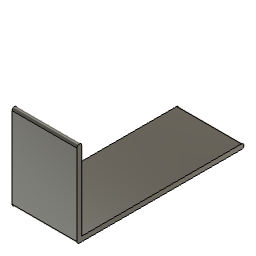
Super Nintendo Bookend (Autodesk Fusion 360 design; units mm, degrees)
Autodesk Fusion 360 part; units mm, degrees
sketch "Sketch1" plane through (0, 0, 0) normal (0, 0, 1) x (1, 0, 0)
  line L0 (0, 0) -> (40, 0)
  line L1 (40, 0) -> (40, 100)
  line L2 (40, 100) -> (0, 100)
  line L3 (0, 100) -> (0, 0)
  line L4 (0, 0) -> (40, 0)
  line L5 (40, 0) -> (40, -3)
  line L6 (40, -3) -> (0, -3)
  line L7 (0, -3) -> (0, 0)
  dimension "d1" = 40
  dimension "d2" = 100
  dimension "d3" = 3
  constraint horizontal L0
  constraint vertical L1
  constraint horizontal L2
  constraint vertical L3
  constraint coincident L0.start L3.end
  constraint horizontal L4
  constraint vertical L5
  constraint horizontal L6
  constraint vertical L7
  measures "d1" distance of L0.start L0.end
  measures "d2" distance of L0.start L2.end
  measures "d3" distance of L0.start L6.end
extrude "Extrude1" add sketch "Sketch1" along normal blind 3 contours L0 L1 L2 L3 L4
extrude "Extrude2" add sketch "Sketch1" along normal blind 53 contours L0 L4 L5 L6 L7
sketch "Sketch2" plane through (0, 0, 0) normal (0, 0, -1) x (1, 0, 0)
  line L0 (0, 3) -> (0, -100)
  line L1 (0, -100) -> (40, -100)
  line L2 (40, -100) -> (40, 3)
  line L3 (40, 3) -> (0, 3)
  line L4 (24.7693, -53.3473) -> (24.431, -53.3473)
  spline S0 degree 3 poles (24.431, -53.3473) (24.2139, -53.3473) (24.1606, -53.2593) (24.1978, -53.0849) knots 0 0 0 0 1 1 1 1
  line L5 (24.1978, -53.0849) -> (24.5069, -51.627)
  spline S1 degree 3 poles (24.5069, -51.627) (24.5472, -51.4375) (24.6658, -51.3707) (24.7869, -51.3707) knots 0 0 0 0 1 1 1 1
  line L6 (24.7869, -51.3707) -> (25.1077, -51.3707)
  spline S2 degree 3 poles (25.1077, -51.3707) (25.2147, -51.3707) (25.2409, -51.4245) (25.2243, -51.5104) knots 0 0 0 0 1 1 1 1
  line L7 (25.2243, -51.5104) -> (24.8804, -53.3006)
  spline S3 degree 3 poles (24.8804, -53.3006) (24.8729, -53.3388) (24.8277, -53.3473) (24.7693, -53.3473) knots 0 0 0 0 1 1 1 1
  line L8 (29.44, -53.3473) -> (29.0786, -53.3473)
  spline S4 degree 3 poles (29.0786, -53.3473) (28.8549, -53.3473) (28.8282, -53.1648) (28.8453, -53.0849) knots 0 0 0 0 1 1 1 1
  line L9 (28.8453, -53.0849) -> (29.1545, -51.621)
  spline S5 degree 3 poles (29.1545, -51.621) (29.1912, -51.4466) (29.2711, -51.3702) (29.347, -51.3702) knots 0 0 0 0 1 1 1 1
  line L10 (29.347, -51.3702) -> (29.7844, -51.3702)
  spline S6 degree 3 poles (29.7844, -51.3702) (29.8879, -51.3702) (29.9186, -51.4199) (29.901, -51.5099) knots 0 0 0 0 1 1 1 1
  line L11 (29.901, -51.5099) -> (29.5511, -53.3001)
  spline S7 degree 3 poles (29.5511, -53.3001) (29.5431, -53.3408) (29.4802, -53.3468) (29.44, -53.3473) knots 0 0 0 0 1 1 1 1
  spline S8 degree 3 poles (3.9225, -53.3709) (3.7023, -53.3709) (3.5566, -53.194) (3.5958, -52.9743) knots 0 0 0 0 1 1 1 1
  line L12 (3.5958, -52.9743) -> (4.2955, -49.0964)
  spline S9 degree 3 poles (4.2955, -49.0964) (4.3353, -48.8772) (4.5363, -48.6942) (4.756, -48.6942) knots 0 0 0 0 1 1 1 1
  spline S10 degree 3 poles (4.756, -48.6942) (4.9762, -48.6942) (5.0692, -48.8767) (5.03, -49.0964) knots 0 0 0 0 1 1 1 1
  line L13 (5.03, -49.0964) -> (4.3363, -52.9743)
  spline S11 degree 3 poles (4.3363, -52.9743) (4.2945, -53.2071) (4.1498, -53.3709) (3.9225, -53.3709) knots 0 0 0 0 1 1 1 1
  line L14 (6.9488, -53.3709) -> (6.605, -53.3709)
  spline S12 degree 3 poles (6.605, -53.3709) (6.3848, -53.3709) (6.231, -53.194) (6.2727, -52.9743) knots 0 0 0 0 1 1 1 1
  line L15 (6.2727, -52.9743) -> (7.0077, -49.0964)
  spline S13 degree 3 poles (7.0077, -49.0964) (7.0494, -48.8767) (7.26, -48.6942) (7.4802, -48.6942) knots 0 0 0 0 1 1 1 1
  line L16 (7.4802, -48.6942) -> (7.8185, -48.6942)
  line L17 (7.8185, -48.6942) -> (6.9498, -53.3709)
  line L18 (6.9498, -53.3709) -> (6.9488, -53.3709)
  spline S14 degree 3 poles (4.383, -54.0531) (4.7027, -54.0531) (5.0084, -53.7902) (5.0652, -53.4639) knots 0 0 0 0 1 1 1 1
  line L19 (5.0652, -53.4639) -> (5.8992, -48.6766)
  spline S15 degree 3 poles (5.8992, -48.6766) (5.9525, -48.371) (5.7509, -48.1287) (5.4442, -48.1287) knots 0 0 0 0 1 1 1 1
  line L20 (5.4442, -48.1287) -> (4.2136, -48.1287)
  spline S16 degree 3 poles (4.2136, -48.1287) (3.9049, -48.1287) (3.6063, -48.3715) (3.549, -48.6766) knots 0 0 0 0 1 1 1 1
  line L21 (3.549, -48.6766) -> (2.6452, -53.4639)
  spline S17 degree 3 poles (2.6452, -53.4639) (2.5838, -53.7902) (2.7924, -54.0531) (3.1122, -54.0531) knots 0 0 0 0 1 1 1 1
  line L22 (3.1122, -54.0531) -> (4.383, -54.0531)
  line L23 (7.5848, -54.0531) -> (8.7103, -48.1287)
  line L24 (8.7103, -48.1287) -> (7.0077, -48.1287)
  spline S18 degree 3 poles (7.0077, -48.1287) (6.6985, -48.1287) (6.4004, -48.3715) (6.3431, -48.6766) knots 0 0 0 0 1 1 1 1
  line L25 (6.3431, -48.6766) -> (5.4392, -53.4639)
  spline S19 degree 3 poles (5.4392, -53.4639) (5.3769, -53.7907) (5.5855, -54.0531) (5.9052, -54.0531) knots 0 0 0 0 1 1 1 1
  line L26 (5.9052, -54.0531) -> (7.5848, -54.0531)
  line L27 (10.5528, -54.0531) -> (11.6783, -48.1287)
  line L28 (11.6783, -48.1287) -> (10.8152, -48.1287)
  line L29 (10.8152, -48.1287) -> (10.1214, -51.5632)
  line L30 (10.1214, -51.5632) -> (9.8475, -48.1287)
  line L31 (9.8475, -48.1287) -> (9.1009, -48.1287)
  line L32 (9.1009, -48.1287) -> (7.9754, -54.0531)
  line L33 (7.9754, -54.0531) -> (8.8385, -54.0531)
  line L34 (8.8385, -54.0531) -> (9.4156, -50.9569)
  line L35 (9.4156, -50.9569) -> (9.8007, -54.0531)
  line L36 (9.8007, -54.0531) -> (10.5528, -54.0531)
  line L37 (12.448, -54.0531) -> (13.6143, -48.1287)
  line L38 (13.6143, -48.1287) -> (11.9754, -48.1287)
  line L39 (11.9754, -48.1287) -> (11.8181, -48.8637)
  line L40 (11.8181, -48.8637) -> (12.6973, -48.8637)
  line L41 (12.6973, -48.8637) -> (12.3022, -50.8639)
  line L42 (12.3022, -50.8639) -> (11.4742, -50.8639)
  line L43 (11.4742, -50.8639) -> (11.3576, -51.4823)
  line L44 (11.3576, -51.4823) -> (12.1856, -51.4823)
  line L45 (12.1856, -51.4823) -> (11.8241, -53.3192)
  line L46 (11.8241, -53.3192) -> (10.9961, -53.3192)
  line L47 (10.9961, -53.3192) -> (10.8649, -54.0531)
  line L48 (10.8649, -54.0531) -> (12.448, -54.0531)
  line L49 (14.5005, -54.0531) -> (14.6403, -53.3182)
  line L50 (14.6403, -53.3182) -> (14.1738, -53.3182)
  line L51 (14.1738, -53.3182) -> (15.0952, -48.1282)
  line L52 (15.0952, -48.1282) -> (14.2436, -48.1282)
  line L53 (14.2436, -48.1282) -> (13.3046, -53.3182)
  line L54 (13.3046, -53.3182) -> (12.8808, -53.3182)
  line L55 (12.8808, -53.3182) -> (12.7395, -54.0531)
  line L56 (12.7395, -54.0531) -> (14.5005, -54.0531)
  line L57 (17.3926, -54.0531) -> (18.5182, -48.1287)
  line L58 (18.5182, -48.1287) -> (17.655, -48.1287)
  line L59 (17.655, -48.1287) -> (16.9613, -51.5632)
  line L60 (16.9613, -51.5632) -> (16.6873, -48.1287)
  line L61 (16.6873, -48.1287) -> (15.9408, -48.1287)
  line L62 (15.9408, -48.1287) -> (14.8152, -54.0531)
  line L63 (14.8152, -54.0531) -> (15.6784, -54.0531)
  line L64 (15.6784, -54.0531) -> (16.2555, -50.9569)
  line L65 (16.2555, -50.9569) -> (16.6406, -54.0531)
  line L66 (16.6406, -54.0531) -> (17.3926, -54.0531)
  line L67 (18.5297, -54.0531) -> (19.6553, -48.1287)
  line L68 (19.6553, -48.1287) -> (18.9088, -48.1287)
  line L69 (18.9088, -48.1287) -> (17.7837, -54.0531)
  line L70 (17.7837, -54.0531) -> (18.5297, -54.0531)
  line L71 (21.4922, -54.0531) -> (22.6178, -48.1287)
  line L72 (22.6178, -48.1287) -> (21.7606, -48.1287)
  line L73 (21.7606, -48.1287) -> (21.0669, -51.5632)
  line L74 (21.0669, -51.5632) -> (20.7929, -48.1287)
  line L75 (20.7929, -48.1287) -> (20.0464, -48.1287)
  line L76 (20.0464, -48.1287) -> (18.9208, -54.0531)
  line L77 (18.9208, -54.0531) -> (19.778, -54.0531)
  line L78 (19.778, -54.0531) -> (20.3611, -50.9569)
  line L79 (20.3611, -50.9569) -> (20.7457, -54.0531)
  line L80 (20.7457, -54.0531) -> (21.4922, -54.0531)
  line L81 (25.4867, -54.0531) -> (26.6062, -48.1287)
  line L82 (26.6062, -48.1287) -> (25.8597, -48.1287)
  line L83 (25.8597, -48.1287) -> (25.3525, -50.8111)
  line L84 (25.3525, -50.8111) -> (24.8216, -50.8111)
  spline S20 degree 3 poles (24.8216, -50.8111) (24.698, -50.8111) (24.6487, -50.6392) (24.7166, -50.2803) knots 0 0 0 0 1 1 1 1
  line L85 (24.7166, -50.2803) -> (25.1248, -48.1287)
  line L86 (25.1248, -48.1287) -> (24.3782, -48.1287)
  line L87 (24.3782, -48.1287) -> (23.9585, -50.4145)
  spline S21 degree 3 poles (23.9585, -50.4145) (23.9032, -50.7141) (24.147, -50.8539) (24.4019, -50.9102) knots 0 0 0 0 1 1 1 1
  spline S22 degree 3 poles (24.4019, -50.9102) (24.1882, -50.9941) (23.7866, -51.1334) (23.7428, -51.3591) knots 0 0 0 0 1 1 1 1
  line L88 (23.7428, -51.3591) -> (23.3346, -53.4639)
  spline S23 degree 3 poles (23.3346, -53.4639) (23.2718, -53.7907) (23.4814, -54.0531) (23.8011, -54.0531) knots 0 0 0 0 1 1 1 1
  line L89 (23.8011, -54.0531) -> (25.4867, -54.0531)
  line L90 (27.4925, -54.0531) -> (28.6588, -48.1287)
  line L91 (28.6588, -48.1287) -> (27.0154, -48.1287)
  line L92 (27.0154, -48.1287) -> (26.8626, -48.8637)
  line L93 (26.8626, -48.8637) -> (27.7409, -48.8637)
  line L94 (27.7409, -48.8637) -> (27.3523, -50.8639)
  line L95 (27.3523, -50.8639) -> (26.5243, -50.8639)
  line L96 (26.5243, -50.8639) -> (26.4077, -51.4823)
  line L97 (26.4077, -51.4823) -> (27.2356, -51.4823)
  line L98 (27.2356, -51.4823) -> (26.8682, -53.3192)
  line L99 (26.8682, -53.3192) -> (26.0402, -53.3192)
  line L100 (26.0402, -53.3192) -> (25.9035, -54.0531)
  line L101 (25.9035, -54.0531) -> (27.4925, -54.0531)
  line L102 (30.1574, -54.0531) -> (31.2829, -48.1287)
  line L103 (31.2829, -48.1287) -> (30.5364, -48.1287)
  line L104 (30.5364, -48.1287) -> (30.0232, -50.8111)
  line L105 (30.0232, -50.8111) -> (29.1183, -50.8111)
  spline S24 degree 3 poles (29.1183, -50.8111) (28.8091, -50.8111) (28.5246, -51.0575) (28.4592, -51.3591) knots 0 0 0 0 1 1 1 1
  line L106 (28.4592, -51.3591) -> (28.0053, -53.4639)
  spline S25 degree 3 poles (28.0053, -53.4639) (27.9359, -53.7892) (28.1521, -54.0531) (28.4723, -54.0531) knots 0 0 0 0 1 1 1 1
  line L107 (28.4723, -54.0531) -> (30.1574, -54.0531)
  line L108 (32.8398, -54.0531) -> (33.8307, -48.6766)
  spline S26 degree 3 poles (33.8307, -48.6766) (33.887, -48.3715) (33.6773, -48.1287) (33.3702, -48.1287) knots 0 0 0 0 1 1 1 1
  line L109 (33.3702, -48.1287) -> (32.2562, -48.1287)
  spline S27 degree 3 poles (32.2562, -48.1287) (31.9475, -48.1287) (31.6514, -48.372) (31.5916, -48.6766) knots 0 0 0 0 1 1 1 1
  line L110 (31.5916, -48.6766) -> (30.5364, -54.0531)
  line L111 (30.5364, -54.0531) -> (31.2362, -54.0531)
  line L112 (31.2362, -54.0531) -> (32.2848, -48.8285)
  spline S28 degree 3 poles (32.2848, -48.8285) (32.2999, -48.7531) (32.3723, -48.6887) (32.4482, -48.6887) knots 0 0 0 0 1 1 1 1
  line L113 (32.4482, -48.6887) -> (33.0022, -48.6887)
  spline S29 degree 3 poles (33.0022, -48.6887) (33.0796, -48.6887) (33.1339, -48.7526) (33.1188, -48.8285) knots 0 0 0 0 1 1 1 1
  line L114 (33.1188, -48.8285) -> (32.0933, -54.0531)
  line L115 (32.0933, -54.0531) -> (32.8398, -54.0531)
  spline S30 degree 3 poles (34.9859, -54.0531) (35.3056, -54.0531) (35.6087, -53.7887) (35.6741, -53.4639) knots 0 0 0 0 1 1 1 1
  line L116 (35.6741, -53.4639) -> (35.9018, -52.3328)
  spline S31 degree 3 poles (35.9018, -52.3328) (35.93, -52.1931) (35.8747, -52.091) (35.8435, -51.9598) knots 0 0 0 0 1 1 1 1
  spline S32 degree 3 poles (35.8435, -51.9598) (35.7696, -51.6497) (34.7325, -50.1913) (34.7707, -49.9711) knots 0 0 0 0 1 1 1 1
  line L117 (34.7707, -49.9711) -> (34.9225, -49.0964)
  spline S33 degree 3 poles (34.9225, -49.0964) (34.9608, -48.8762) (35.1106, -48.6998) (35.3307, -48.6998) knots 0 0 0 0 1 1 1 1
  spline S34 degree 3 poles (35.3307, -48.6998) (35.5509, -48.6998) (35.7033, -48.8762) (35.663, -49.0964) knots 0 0 0 0 1 1 1 1
  line L118 (35.663, -49.0964) -> (35.465, -50.1813)
  line L119 (35.465, -50.1813) -> (36.2457, -50.1813)
  line L120 (36.2457, -50.1813) -> (36.5081, -48.6766)
  spline S35 degree 3 poles (36.5081, -48.6766) (36.5614, -48.371) (36.3548, -48.1287) (36.0476, -48.1287) knots 0 0 0 0 1 1 1 1
  line L121 (36.0476, -48.1287) -> (34.9336, -48.1287)
  spline S36 degree 3 poles (34.9336, -48.1287) (34.6249, -48.1287) (34.3314, -48.3715) (34.2746, -48.6766) knots 0 0 0 0 1 1 1 1
  spline S37 degree 3 poles (34.2746, -48.6766) (34.2228, -48.9577) (33.989, -50.0817) (33.989, -50.1813) knots 0 0 0 0 1 1 1 1
  spline S38 degree 3 poles (33.989, -50.1813) (33.989, -50.2381) (34.0086, -50.2763) (34.0182, -50.2919) knots 0 0 0 0 1 1 1 1
  line L122 (34.0182, -50.2919) -> (35.0447, -52.0006)
  spline S39 degree 3 poles (35.0447, -52.0006) (35.1096, -52.1086) (35.1191, -52.177) (35.1206, -52.269) knots 0 0 0 0 1 1 1 1
  spline S40 degree 3 poles (35.1206, -52.269) (35.1221, -52.3605) (35.0326, -52.7732) (34.998, -52.9748) knots 0 0 0 0 1 1 1 1
  spline S41 degree 3 poles (34.998, -52.9748) (34.9603, -53.195) (34.7516, -53.3714) (34.5314, -53.3714) knots 0 0 0 0 1 1 1 1
  spline S42 degree 3 poles (34.5314, -53.3714) (34.3113, -53.3714) (34.1836, -53.194) (34.2278, -52.9748) knots 0 0 0 0 1 1 1 1
  line L123 (34.2278, -52.9748) -> (34.4264, -52.0011)
  line L124 (34.4264, -52.0011) -> (33.6391, -52.0011)
  line L125 (33.6391, -52.0011) -> (33.3652, -53.4649)
  spline S43 degree 3 poles (33.3652, -53.4649) (33.3038, -53.7902) (33.5114, -54.0531) (33.8312, -54.0531) knots 0 0 0 0 1 1 1 1
  line L126 (33.8312, -54.0531) -> (34.9859, -54.0531)
  line L127 (36.6418, -47.6154) -> (36.6418, -45.6735)
  line L128 (36.6418, -45.6735) -> (3.357, -45.6735)
  line L129 (3.357, -45.6735) -> (3.357, -47.6154)
  line L130 (3.357, -47.6154) -> (36.6418, -47.6154)
  line L131 (35.9189, -47.3646) -> (35.5751, -47.3646)
  line L132 (35.5751, -47.3646) -> (35.5982, -47.2012)
  line L133 (35.5982, -47.2012) -> (35.7847, -47.2012)
  line L134 (35.7847, -47.2012) -> (35.8606, -46.793)
  line L135 (35.8606, -46.793) -> (35.6796, -46.793)
  line L136 (35.6796, -46.793) -> (35.7028, -46.6527)
  line L137 (35.7028, -46.6527) -> (35.8893, -46.6527)
  line L138 (35.8893, -46.6527) -> (35.9591, -46.2099)
  line L139 (35.9591, -46.2099) -> (35.7782, -46.2099)
  line L140 (35.7782, -46.2099) -> (35.8073, -46.0465)
  line L141 (35.8073, -46.0465) -> (36.1803, -46.0465)
  line L142 (36.1803, -46.0465) -> (35.9179, -47.3641)
  line L143 (35.9179, -47.3641) -> (35.9189, -47.3646)
  line L144 (34.3092, -47.3646) -> (34.1459, -47.3646)
  line L145 (34.1459, -47.3646) -> (34.0584, -46.6764)
  line L146 (34.0584, -46.6764) -> (33.9302, -47.3646)
  line L147 (33.9302, -47.3646) -> (33.7377, -47.3646)
  line L148 (33.7377, -47.3646) -> (33.9885, -46.047)
  line L149 (33.9885, -46.047) -> (34.1519, -46.047)
  line L150 (34.1519, -46.047) -> (34.2162, -46.8111)
  line L151 (34.2162, -46.8111) -> (34.3681, -46.047)
  line L152 (34.3681, -46.047) -> (34.5606, -46.047)
  line L153 (34.5606, -46.047) -> (34.3092, -47.3646)
  line L154 (32.5598, -47.3646) -> (32.1747, -47.3646)
  line L155 (32.1747, -47.3646) -> (32.1979, -47.2012)
  line L156 (32.1979, -47.2012) -> (32.2969, -47.2012)
  line L157 (32.2969, -47.2012) -> (32.507, -46.0465)
  line L158 (32.507, -46.0465) -> (32.6935, -46.0465)
  line L159 (32.6935, -46.0465) -> (32.4894, -47.2012)
  line L160 (32.4894, -47.2012) -> (32.5945, -47.2012)
  line L161 (32.5945, -47.2012) -> (32.5598, -47.3646)
  line L162 (30.8632, -47.3646) -> (30.5133, -47.3646)
  line L163 (30.5133, -47.3646) -> (30.5425, -47.2012)
  line L164 (30.5425, -47.2012) -> (30.7234, -47.2012)
  line L165 (30.7234, -47.2012) -> (30.8049, -46.793)
  line L166 (30.8049, -46.793) -> (30.6239, -46.793)
  line L167 (30.6239, -46.793) -> (30.647, -46.6527)
  line L168 (30.647, -46.6527) -> (30.828, -46.6527)
  line L169 (30.828, -46.6527) -> (30.9145, -46.2099)
  line L170 (30.9145, -46.2099) -> (30.7229, -46.2099)
  line L171 (30.7229, -46.2099) -> (30.746, -46.0465)
  line L172 (30.746, -46.0465) -> (31.1191, -46.0465)
  line L173 (31.1191, -46.0465) -> (30.8632, -47.3646)
  line L174 (29.2188, -47.3646) -> (28.8458, -47.3646)
  spline S44 degree 3 poles (28.8458, -47.3646) (28.7764, -47.3646) (28.7332, -47.3032) (28.7468, -47.2304) knots 0 0 0 0 1 1 1 1
  line L175 (28.7468, -47.2304) -> (28.8342, -46.7638)
  spline S45 degree 3 poles (28.8342, -46.7638) (28.8438, -46.7131) (28.9328, -46.6718) (28.98, -46.6527) knots 0 0 0 0 1 1 1 1
  spline S46 degree 3 poles (28.98, -46.6527) (28.9142, -46.6527) (28.8709, -46.6206) (28.881, -46.5653) knots 0 0 0 0 1 1 1 1
  line L176 (28.881, -46.5653) -> (28.9745, -46.0465)
  line L177 (28.9745, -46.0465) -> (29.1439, -46.0465)
  line L178 (29.1439, -46.0465) -> (29.0504, -46.5246)
  spline S47 degree 3 poles (29.0504, -46.5246) (29.0424, -46.5663) (29.0358, -46.6412) (29.0735, -46.6412) knots 0 0 0 0 1 1 1 1
  line L179 (29.0735, -46.6412) -> (29.1902, -46.6412)
  line L180 (29.1902, -46.6412) -> (29.3008, -46.0465)
  line L181 (29.3008, -46.0465) -> (29.4697, -46.0465)
  line L182 (29.4697, -46.0465) -> (29.2188, -47.3646)
  line L183 (27.5508, -47.3646) -> (27.1602, -47.3646)
  line L184 (27.1602, -47.3646) -> (27.1834, -47.2012)
  line L185 (27.1834, -47.2012) -> (27.2824, -47.2012)
  line L186 (27.2824, -47.2012) -> (27.4925, -46.0465)
  line L187 (27.4925, -46.0465) -> (27.679, -46.0465)
  line L188 (27.679, -46.0465) -> (27.4749, -47.2012)
  line L189 (27.4749, -47.2012) -> (27.58, -47.2012)
  line L190 (27.58, -47.2012) -> (27.5508, -47.3646)
  line L191 (25.5948, -47.3646) -> (25.4239, -47.3646)
  line L192 (25.4239, -47.3646) -> (25.4832, -46.047)
  line L193 (25.4832, -46.047) -> (25.6798, -46.047)
  line L194 (25.6798, -46.047) -> (25.6506, -46.3501)
  line L195 (25.6506, -46.3501) -> (25.7848, -46.3501)
  line L196 (25.7848, -46.3501) -> (25.8778, -46.047)
  line L197 (25.8778, -46.047) -> (26.0688, -46.047)
  line L198 (26.0688, -46.047) -> (25.5958, -47.3646)
  line L199 (25.5958, -47.3646) -> (25.5948, -47.3646)
  line L200 (24.058, -47.3646) -> (23.8891, -47.3646)
  line L201 (23.8891, -47.3646) -> (24.14, -46.047)
  line L202 (24.14, -46.047) -> (24.3033, -46.047)
  line L203 (24.3033, -46.047) -> (24.058, -47.3646)
  line L204 (22.5534, -47.3646) -> (22.39, -47.3646)
  line L205 (22.39, -47.3646) -> (22.3026, -46.6764)
  line L206 (22.3026, -46.6764) -> (22.1744, -47.3646)
  line L207 (22.1744, -47.3646) -> (21.9879, -47.3646)
  line L208 (21.9879, -47.3646) -> (22.2327, -46.047)
  line L209 (22.2327, -46.047) -> (22.4016, -46.047)
  line L210 (22.4016, -46.047) -> (22.4745, -46.8111)
  line L211 (22.4745, -46.8111) -> (22.6117, -46.047)
  line L212 (22.6117, -46.047) -> (22.8043, -46.047)
  line L213 (22.8043, -46.047) -> (22.5534, -47.3646)
  line L214 (20.6235, -47.3646) -> (20.4078, -47.3646)
  line L215 (20.4078, -47.3646) -> (20.3727, -46.6005)
  line L216 (20.3727, -46.6005) -> (20.0379, -47.3646)
  line L217 (20.0379, -47.3646) -> (19.8292, -47.3646)
  line L218 (19.8292, -47.3646) -> (20.0519, -46.047)
  line L219 (20.0519, -46.047) -> (20.2153, -46.047)
  line L220 (20.2153, -46.047) -> (20.1102, -46.7407)
  line L221 (20.1102, -46.7407) -> (20.4018, -46.047)
  line L222 (20.4018, -46.047) -> (20.5184, -46.047)
  line L223 (20.5184, -46.047) -> (20.5536, -46.7583)
  line L224 (20.5536, -46.7583) -> (20.6818, -46.047)
  line L225 (20.6818, -46.047) -> (20.8683, -46.047)
  line L226 (20.8683, -46.047) -> (20.6235, -47.3646)
  line L227 (18.5066, -47.3646) -> (18.1572, -47.3646)
  line L228 (18.1572, -47.3646) -> (18.1859, -47.2012)
  line L229 (18.1859, -47.2012) -> (18.3724, -47.2012)
  line L230 (18.3724, -47.2012) -> (18.4483, -46.793)
  line L231 (18.4483, -46.793) -> (18.2673, -46.793)
  line L232 (18.2673, -46.793) -> (18.2904, -46.6527)
  line L233 (18.2904, -46.6527) -> (18.4769, -46.6527)
  line L234 (18.4769, -46.6527) -> (18.5679, -46.2099)
  line L235 (18.5679, -46.2099) -> (18.3658, -46.2099)
  line L236 (18.3658, -46.2099) -> (18.395, -46.0465)
  line L237 (18.395, -46.0465) -> (18.7625, -46.0465)
  line L238 (18.7625, -46.0465) -> (18.5066, -47.3646)
  line L239 (16.8155, -47.3646) -> (16.6521, -47.3646)
  line L240 (16.6521, -47.3646) -> (16.5646, -46.6764)
  line L241 (16.5646, -46.6764) -> (16.4365, -47.3646)
  line L242 (16.4365, -47.3646) -> (16.2499, -47.3646)
  line L243 (16.2499, -47.3646) -> (16.4948, -46.047)
  line L244 (16.4948, -46.047) -> (16.6581, -46.047)
  line L245 (16.6581, -46.047) -> (16.7225, -46.8111)
  line L246 (16.7225, -46.8111) -> (16.8743, -46.047)
  line L247 (16.8743, -46.047) -> (17.0668, -46.047)
  line L248 (17.0668, -46.047) -> (16.8155, -47.3646)
  line L249 (15.0837, -47.3646) -> (14.6931, -47.3646)
  line L250 (14.6931, -47.3646) -> (14.7222, -47.2012)
  line L251 (14.7222, -47.2012) -> (14.8213, -47.2012)
  line L252 (14.8213, -47.2012) -> (15.0254, -46.0465)
  line L253 (15.0254, -46.0465) -> (15.2119, -46.0465)
  line L254 (15.2119, -46.0465) -> (15.0078, -47.2012)
  line L255 (15.0078, -47.2012) -> (15.1128, -47.2012)
  line L256 (15.1128, -47.2012) -> (15.0837, -47.3646)
  line L257 (10.8328, -47.3646) -> (10.6458, -47.3646)
  line L258 (10.6458, -47.3646) -> (10.5834, -46.8629)
  line L259 (10.5834, -46.8629) -> (10.3255, -47.3646)
  line L260 (10.3255, -47.3646) -> (10.1154, -47.3646)
  line L261 (10.1154, -47.3646) -> (10.5467, -46.6005)
  line L262 (10.5467, -46.6005) -> (10.6518, -46.0465)
  line L263 (10.6518, -46.0465) -> (10.8383, -46.0465)
  line L264 (10.8383, -46.0465) -> (10.7222, -46.6412)
  line L265 (10.7222, -46.6412) -> (10.8328, -47.3646)
  line L266 (7.5823, -47.3646) -> (7.1751, -47.3646)
  line L267 (7.1751, -47.3646) -> (7.2057, -47.2012)
  line L268 (7.2057, -47.2012) -> (7.3048, -47.2012)
  line L269 (7.3048, -47.2012) -> (7.5089, -46.0465)
  line L270 (7.5089, -46.0465) -> (7.7014, -46.0465)
  line L271 (7.7014, -46.0465) -> (7.4973, -47.2012)
  line L272 (7.4973, -47.2012) -> (7.6124, -47.2012)
  line L273 (7.6124, -47.2012) -> (7.5823, -47.3646)
  line L274 (6.0374, -47.3646) -> (5.6875, -47.3646)
  line L275 (5.6875, -47.3646) -> (5.7187, -47.2012)
  line L276 (5.7187, -47.2012) -> (5.8997, -47.2012)
  line L277 (5.8997, -47.2012) -> (5.9811, -46.787)
  line L278 (5.9811, -46.787) -> (5.7946, -46.787)
  line L279 (5.7946, -46.787) -> (5.8182, -46.6527)
  line L280 (5.8182, -46.6527) -> (6.0042, -46.6527)
  line L281 (6.0042, -46.6527) -> (6.0927, -46.2094)
  line L282 (6.0927, -46.2094) -> (5.8942, -46.2094)
  line L283 (5.8942, -46.2094) -> (5.9223, -46.046)
  line L284 (5.9223, -46.046) -> (6.2953, -46.046)
  line L285 (6.2953, -46.046) -> (6.0369, -47.3636)
  line L286 (6.0369, -47.3636) -> (6.0374, -47.3646)
  line L287 (4.5992, -47.3646) -> (4.3835, -47.3646)
  line L288 (4.3835, -47.3646) -> (4.3483, -46.6005)
  line L289 (4.3483, -46.6005) -> (4.016, -47.3646)
  line L290 (4.016, -47.3646) -> (3.8059, -47.3646)
  line L291 (3.8059, -47.3646) -> (4.0276, -46.047)
  line L292 (4.0276, -46.047) -> (4.191, -46.047)
  line L293 (4.191, -46.047) -> (4.0859, -46.7407)
  line L294 (4.0859, -46.7407) -> (4.3775, -46.047)
  line L295 (4.3775, -46.047) -> (4.4941, -46.047)
  line L296 (4.4941, -46.047) -> (4.5293, -46.7583)
  line L297 (4.5293, -46.7583) -> (4.6575, -46.047)
  line L298 (4.6575, -46.047) -> (4.85, -46.047)
  line L299 (4.85, -46.047) -> (4.5992, -47.3646)
  line L300 (12.1448, -47.3591) -> (11.8885, -47.3591)
  spline S48 degree 3 poles (11.8885, -47.3591) (11.8191, -47.3591) (11.7718, -47.3038) (11.7834, -47.2309) knots 0 0 0 0 1 1 1 1
  line L301 (11.7834, -47.2309) -> (11.8352, -46.9041)
  line L302 (11.8352, -46.9041) -> (12.0096, -46.9041)
  line L303 (12.0096, -46.9041) -> (11.9704, -47.1198)
  spline S49 degree 3 poles (11.9704, -47.1198) (11.9613, -47.1685) (11.991, -47.2072) (12.0403, -47.2072) knots 0 0 0 0 1 1 1 1
  spline S50 degree 3 poles (12.0403, -47.2072) (12.0895, -47.2072) (12.1363, -47.1685) (12.1453, -47.1198) knots 0 0 0 0 1 1 1 1
  line L304 (12.1453, -47.1198) -> (12.1745, -46.9624)
  spline S51 degree 3 poles (12.1745, -46.9624) (12.1765, -46.9519) (12.1619, -46.9116) (12.1569, -46.9041) knots 0 0 0 0 1 1 1 1
  line L305 (12.1569, -46.9041) -> (11.9121, -46.5251)
  spline S52 degree 3 poles (11.9121, -46.5251) (11.9045, -46.5135) (11.9055, -46.5065) (11.906, -46.5019) knots 0 0 0 0 1 1 1 1
  line L306 (11.906, -46.5019) -> (11.9704, -46.1696)
  spline S53 degree 3 poles (11.9704, -46.1696) (11.9835, -46.1033) (12.0478, -46.047) (12.1162, -46.047) knots 0 0 0 0 1 1 1 1
  line L307 (12.1162, -46.047) -> (12.3781, -46.047)
  spline S54 degree 3 poles (12.3781, -46.047) (12.446, -46.047) (12.4892, -46.1028) (12.4771, -46.1696) knots 0 0 0 0 1 1 1 1
  line L308 (12.4771, -46.1696) -> (12.4188, -46.5019)
  line L309 (12.4188, -46.5019) -> (12.2499, -46.5019)
  line L310 (12.2499, -46.5019) -> (12.2906, -46.2626)
  spline S55 degree 3 poles (12.2906, -46.2626) (12.2992, -46.2139) (12.27, -46.1691) (12.2207, -46.1691) knots 0 0 0 0 1 1 1 1
  spline S56 degree 3 poles (12.2207, -46.1691) (12.1715, -46.1691) (12.1247, -46.2134) (12.1157, -46.2626) knots 0 0 0 0 1 1 1 1
  line L311 (12.1157, -46.2626) -> (12.0805, -46.4552)
  line L312 (12.0805, -46.4552) -> (12.3313, -46.8986)
  spline S57 degree 3 poles (12.3313, -46.8986) (12.3374, -46.9091) (12.3489, -46.9488) (12.3429, -46.98) knots 0 0 0 0 1 1 1 1
  line L313 (12.3429, -46.98) -> (12.2961, -47.2309)
  spline S58 degree 3 poles (12.2961, -47.2309) (12.2806, -47.3153) (12.2449, -47.3591) (12.1448, -47.3591) knots 0 0 0 0 1 1 1 1
  line L314 (8.8963, -47.3591) -> (8.64, -47.3591)
  spline S59 degree 3 poles (8.64, -47.3591) (8.5706, -47.3591) (8.5233, -47.3038) (8.5349, -47.2309) knots 0 0 0 0 1 1 1 1
  line L315 (8.5349, -47.2309) -> (8.5867, -46.9041)
  line L316 (8.5867, -46.9041) -> (8.7611, -46.9041)
  line L317 (8.7611, -46.9041) -> (8.7214, -47.1198)
  spline S60 degree 3 poles (8.7214, -47.1198) (8.7123, -47.1685) (8.742, -47.2072) (8.7913, -47.2072) knots 0 0 0 0 1 1 1 1
  spline S61 degree 3 poles (8.7913, -47.2072) (8.8405, -47.2072) (8.8873, -47.1685) (8.8963, -47.1198) knots 0 0 0 0 1 1 1 1
  line L318 (8.8963, -47.1198) -> (8.9255, -46.9624)
  spline S62 degree 3 poles (8.9255, -46.9624) (8.9275, -46.9519) (8.9129, -46.9116) (8.9079, -46.9041) knots 0 0 0 0 1 1 1 1
  line L319 (8.9079, -46.9041) -> (8.6631, -46.5251)
  spline S63 degree 3 poles (8.6631, -46.5251) (8.6555, -46.5135) (8.656, -46.5065) (8.657, -46.5019) knots 0 0 0 0 1 1 1 1
  line L320 (8.657, -46.5019) -> (8.7214, -46.1696)
  spline S64 degree 3 poles (8.7214, -46.1696) (8.7345, -46.1033) (8.7988, -46.047) (8.8672, -46.047) knots 0 0 0 0 1 1 1 1
  line L321 (8.8672, -46.047) -> (9.1291, -46.047)
  spline S65 degree 3 poles (9.1291, -46.047) (9.197, -46.047) (9.2402, -46.1028) (9.2281, -46.1696) knots 0 0 0 0 1 1 1 1
  line L322 (9.2281, -46.1696) -> (9.1698, -46.5019)
  line L323 (9.1698, -46.5019) -> (9.0009, -46.5019)
  line L324 (9.0009, -46.5019) -> (9.0416, -46.2626)
  spline S66 degree 3 poles (9.0416, -46.2626) (9.0502, -46.2139) (9.021, -46.1691) (8.9717, -46.1691) knots 0 0 0 0 1 1 1 1
  spline S67 degree 3 poles (8.9717, -46.1691) (8.9225, -46.1691) (8.8757, -46.2134) (8.8667, -46.2626) knots 0 0 0 0 1 1 1 1
  line L325 (8.8667, -46.2626) -> (8.8315, -46.4552)
  line L326 (8.8315, -46.4552) -> (9.0823, -46.8986)
  spline S68 degree 3 poles (9.0823, -46.8986) (9.0884, -46.9091) (9.0999, -46.9488) (9.0939, -46.98) knots 0 0 0 0 1 1 1 1
  line L327 (9.0939, -46.98) -> (9.0472, -47.2309)
  spline S69 degree 3 poles (9.0472, -47.2309) (9.0316, -47.3153) (8.9964, -47.3591) (8.8953, -47.3591) knots 0 0 0 0 1 1 1 1
  line L328 (8.8953, -47.3591) -> (8.8963, -47.3591)
  spline S70 degree 3 poles (29.061, -47.2072) (29.07, -47.2072) (29.0826, -47.2047) (29.0841, -47.1957) knots 0 0 0 0 1 1 1 1
  line L329 (29.0841, -47.1957) -> (29.16, -46.7935)
  spline S71 degree 3 poles (29.16, -46.7935) (29.1625, -46.7809) (29.151, -46.7704) (29.1369, -46.7704) knots 0 0 0 0 1 1 1 1
  line L330 (29.1369, -46.7704) -> (29.067, -46.7704)
  spline S72 degree 3 poles (29.067, -46.7704) (29.0218, -46.7704) (29.0062, -46.8056) (29.0027, -46.8227) knots 0 0 0 0 1 1 1 1
  line L331 (29.0027, -46.8227) -> (28.9383, -47.1494)
  spline S73 degree 3 poles (28.9383, -47.1494) (28.9348, -47.168) (28.9413, -47.2077) (28.9851, -47.2077) knots 0 0 0 0 1 1 1 1
  line L332 (28.9851, -47.2077) -> (29.061, -47.2072)
  line L333 (25.5983, -46.9041) -> (25.7315, -46.4778)
  line L334 (25.7315, -46.4778) -> (25.638, -46.4778)
  line L335 (25.638, -46.4778) -> (25.5983, -46.9041)
extrude "Extrude3" cut sketch "Sketch2" against normal blind 1 contours S14 L19 S15 L20 S16 L21 S17 L22 | L23 L24 S18 L25 S19 L26 | L27 L28 L29 L30 L31 L32 L33 L34 L35 L36 | L37 L38 L39 L40 L41 L42 L43 L44 L45 L46 L47 L48 | L49 L50 L51 L52 L53 L54 L55 L56 | L57 L58 L59 L60 L61 L62 L63 L64 L65 L66 | L67 L68 L69 L70 | L71 L72 L73 L74 L75 L76 L77 L78 L79 L80 | L81 L82 L83 L84 S20 L85 L86 L87 S21 S22 L88 S23 L89 | L90 L91 L92 L93 L94 L95 L96 L97 L98 L99 L100 L101 | L102 L103 L104 L105 S24 L106 S25 L107 | L108 S26 L109 S27 L110 L111 L112 S28 L113 S29 L114 L115 | S30 L116 S31 S32 L117 S33 S34 L118 L119 L120 S35 L121 S36 S37 S38 L122 S39 S40 S41 S42 L123 L124 L125 S43 L126 | L127 L128 L129 L130 | S70 L329 S71 L330 S72 L331 S73 L332 | L333 L334 L335
fillet "Fillet1" radius 1.5 2 edges at (20, 100, 3) (20, 100, 0)
fillet "Fillet2" radius 1.5 3 edges at (20, 0, 53) (20, -3, 0) (20, -3, 53)
